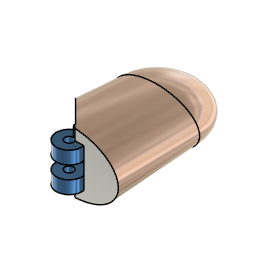
thumb 2 v2 (Autodesk Fusion 360 design; units mm, degrees)
Autodesk Fusion 360 part; units mm, degrees
sketch "base" plane through (0, 0, 0) normal (0, 1, 0) x (1, 0, 0)
  ellipse E0 centre (0, 0) end of major axis (11, 0) minor radius 7
  line L0 (-11, 0) -> (11, 0) construction
  line L1 (0, -7) -> (0, 7) construction
  dimension "d1" = 22
  dimension "d2" = 14
  constraint coincident E0 L0.start
  constraint coincident E0 L0.end
  constraint coincident E0 L1.start
  constraint coincident E0 L1.end
  constraint coincident E0.centre origin
  constraint horizontal L0
  measures "d1" distance of E0
ref_plane "WorkPlane1" through (0, 20, 0) normal (0, 1, 0) x (1, 0, 0)
sketch "top" plane through (0, 20, 0) normal (0, 1, 0) x (1, 0, 0)
  ellipse E0 centre (0, 0) end of major axis (10, 0) minor radius 5.5
  line L0 (-10, 0) -> (10, 0) construction
  line L1 (0, -5.5) -> (0, 5.5) construction
  dimension "d4" = 20
  dimension "d5" = 11
  constraint coincident E0 L0.start
  constraint coincident E0 L0.end
  constraint coincident E0 L1.start
  constraint coincident E0 L1.end
  constraint coincident E0.centre origin
  constraint horizontal L0
  measures "d4" distance of E0
loft "Loft1" add profiles "top", "base" section 1 section 2 makes body 1
sketch "cut" plane through (0, 0, 0) normal (0, 0, 1) x (1, 0, 0)
  line L0 (0, 28) -> (0, 28.5)
  line L1 (0, 0) -> (0, 1)
  line L2 (0, 1) -> (-14.1421, 15.1421)
  line L3 (0, 1) -> (20, 1) construction
  line L4 (-14.1421, 15.1421) -> (-14.1421, 0)
  line L5 (-14.1421, 0) -> (0, 0)
  line L6 (0, 0) -> (0, -0.5)
  line L7 (0, 28) -> (0, 27)
  line L8 (0, 27) -> (20, 27) construction
  line L9 (0, 28) -> (-11.4565, 28)
  line L10 (-11.4565, 28) -> (-14.1421, 12.8579)
  dimension "d6" = 0.5
  dimension "d7" = 1
  dimension "d8" = 135
  dimension "d9" = 20
  dimension "d10" = 0.5
  dimension "d11" = 1
  dimension "d13" = 20
  constraint vertical L0
  constraint coincident L1.start L5.end
  constraint vertical L1
  constraint horizontal L3
  constraint parallel L1 L4
  constraint perpendicular L1 L5
  constraint perpendicular L5 L6
  constraint parallel L0 L7
  constraint horizontal L8
  constraint perpendicular L7 L9
  measures "d6" distance of L0.start L0.end
  measures "d7" distance of L1.start L1.end
  measures "d8" angle of L2 L3
  measures "d9" distance of L1.end L2.end
  measures "d10" distance of L1.start L6.end
  measures "d11" distance of L0.start L7.end
  measures "d13" distance of L7.end L10.end
extrude "Extrude1" cut sketch "cut" along normal mid plane 40 contours L1 L2 L4 L5 L10 bodies 1
sketch "wheel" plane through (0, 0, 0) normal (0, 0, 1) x (1, 0, 0)
  line L0 (0, 0) -> (0, -0.5)
  circle A0 centre (0, -0.5) radius 3
  dimension "d16" = 0.5
  dimension "d17" = 6
  constraint coincident L0.start origin
  constraint vertical L0
  constraint coincident L0.end A0.centre
  measures "d16" distance of L0.start L0.end
  measures "d17" diameter of A0
extrude "Extrude3" cut sketch "wheel" along normal mid plane 3 bodies 1
sketch "lower wheel offset" plane through (0, 0, -1.5) normal (0, 0, 1) x (-1, 0, 0)
  line L0 (0, 0) -> (-2.958, 0)
  arc A0 (-2.958, 0) -> (1.2343, -2.2343) centre (0, 0.5) ccw
  line L1 (0, -1) -> (0, 0)
  circle A1 centre (0, 0.5) radius 3
  line L2 (1.2343, -2.2343) -> (0, -1)
  dimension "d23" = 6
  constraint concentric A0 A1
  measures "d23" diameter of A1
extrude "Extrude4" add sketch "lower wheel offset" against normal blind 3 separate body makes body 2
sketch "lower wheel offset2" plane through (0, 0, 1.5) normal (0, 0, -1) x (1, 0, 0)
  line L0 (2.958, 0) -> (0, 0)
  line L1 (0, 0) -> (0, -1)
  arc A0 (-1.2343, -2.2343) -> (2.958, 0) centre (0, 0.5) ccw
  circle A1 centre (0, 0.5) radius 3
  line L2 (0, -1) -> (-1.2343, -2.2343)
  dimension "d26" = 6
  constraint concentric A0 A1
  measures "d26" diameter of A1
extrude "Extrude5" add sketch "lower wheel offset2" against normal blind 3 separate body makes body 3
sketch "rod cut" plane through (0, 0, 0) normal (0, 0, 1) x (1, 0, 0)
  circle A0 centre (0, -0.5) radius 1
  dimension "d29" = 2
  measures "d29" diameter of A0
copy_body "Body->Comp1" bodies 1 removing the originals makes body 4 in component "index part 1"
copy_body "Body->Comp3" bodies 2 removing the originals makes body 5 in component "lower wheel 1"
copy_body "Body->Comp4" bodies 3 removing the originals makes body 6 in component "lower wheel 2"
sketch "Sketch12" plane through (0, 20, 0) normal (0, 1, 0) x (-1, 0, 0)
  ellipse E0 centre (0, 0) end of major axis (-10, 0) minor radius 5.5
  line L0 (0, -5.5) -> (0, 5.5)
  ellipse E1 centre (0, 0) end of major axis (-10, 0) minor radius 5.5 (0, 5.5) -> (0, -5.5) ccw
  dimension "d46" = 20
  dimension "d47" = 11
  constraint coincident E0.centre E1.centre
  measures "d46" distance of E1
revolve "Revolve1" add sketch "Sketch12" angle 180 about axis through (0, 20, -5.5) along (0, 0, 1) contours E0 L0 E1 bodies 4 in component "index part 1"
extrude "Extrude3'" cut sketch "rod cut" along normal mid plane 40 bodies 4 in component "index part 1"
extrude "Extrude1'" cut sketch "rod cut" along normal mid plane 40 bodies 5 in component "lower wheel 1"
extrude "Extrude1''" cut sketch "rod cut" along normal mid plane 40 bodies 6 in component "lower wheel 2"
combine "Combine1" operation add target body 4 tool bodies 5 6 in component "index part 1"
component "index part 1" placed x (1, 0, 0) y (0, 1, 0) z (0, 0, 1) at (0, 0, 0)
component "lower wheel 1" placed x (1, 0, 0) y (0, 1, 0) z (0, 0, 1) at (0, 0, 0)
component "lower wheel 2" placed x (1, 0, 0) y (0, 1, 0) z (0, 0, 1) at (0, 0, 0)
named bodies: "index part 1", "lower wheel 1", "lower wheel 2"
